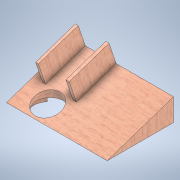
# Autodesk Inventor part: CAP PROCESS SKETCH
Saved by Autodesk Inventor 2021 (Build 250183000, 183)
## iProperties
Created: 2021-07-15
Part Number: CAP PROCESS SKETCH
Material: Generic
Document SubType Name: Modeling
Designer: HP
Density: 1 g/cm^3
Appearance: Plywood - Weathered
Author: HP
Autodesk Inventor part; units mm, degrees
ref_plane "YZ Plane" through (0, 0, 0) normal (1, 0, 0) x (0, 1, 0)
ref_plane "XZ Plane" through (0, 0, 0) normal (0, 1, 0) x (-1, 0, 0)
ref_plane "XY Plane" through (0, 0, 0) normal (0, 0, 1) x (1, 0, 0)
sketch "Sketch1" plane through (0, 0, 0) normal (1, 0, 0) x (0, 1, 0)
  line L0 (0, 0) -> (25.4, 0)
  line L1 (0, 0) -> (0, 75.184)
  line L2 (0, 75.184) -> (25.4, 0)
  dimension "d0" = 25.4
  dimension "d1" = 75.184
  constraints: 6 end point, 1 horizontal, 1 vertical
  measures "d0" distance of L0.start L0.end
  measures "d1" distance of L0.start L1.end
extrude "Extrusion1" add sketch "Sketch1" along normal blind 114.3
sketch "Sketch2" plane through (0, 0, 75.184) normal (0, 0.9473953, 0.320066) x (1, 0, 0)
  circle A0 centre (30.1625, 17.4625) radius 13.4874
  point P0 (0, 71.229)
  dimension "d4" = 26.9748
  constraints: 1 centre point
  measures "d4" diameter of A0
extrude "Extrusion2" add sketch "Sketch2" along normal blind 25.4
sketch "Sketch3" plane through (30.1625, 29.653, 66.7698) normal (0, 0.9473953, 0.320066) x (1, 0, 0)
  circle A0 centre (0, 0) radius 14.9075
  point P0 (-30.1625, 53.7665)
  constraints: 1 centre point
extrude "Extrusion3" cut sketch "Sketch3" against normal blind 76.2
sketch "Sketch4" plane through (0, 0, 0) normal (0, -1, 0) x (1, 0, 0)
  point P0 (0, 0)
sketch "Sketch5" plane through (0, 0, 0) normal (0, -1, 0) x (1, 0, 0)
  arc A0 (42.3045, 45.008) -> (44.45, 66.675) centre (30.1625, 57.15) ccw
  arc A1 (44.3808, 43.1924) -> (47.2504, 67.396) centre (30.1625, 57.15) ccw
  arc A2 (15.875, 66.675) -> (17.0779, 46.0302) centre (30.1625, 57.15) ccw
  arc A3 (13.625, 68.2625) -> (14.8563, 44.3948) centre (30.1625, 57.15) ccw
  line L0 (13.625, 68.2625) -> (15.875, 66.675)
  line L1 (14.8563, 44.3948) -> (17.0779, 46.0302)
  line L2 (44.45, 66.675) -> (47.2504, 67.396)
  line L3 (42.3045, 45.008) -> (44.3808, 43.1924)
  point P0 (0, 0)
  constraints: 8 end point, 8 point on circle, 4 centre point, 3 coincident
extrude "Extrusion4" add sketch "Sketch5" along normal blind 5.08
sketch "Sketch6" plane through (0, 0, 75.184) normal (0, 0.9473953, 0.320066) x (1, 0, 0)
  line L0 (0, 79.3586) -> (114.3, 79.3586) projected
  line L1 (14.2875, 31.75) -> (11.1125, 31.75)
  line L2 (11.1125, 31.75) -> (11.1125, 79.3586)
  line L3 (11.1125, 79.3586) -> (14.2875, 79.3586)
  line L4 (14.2875, 79.3586) -> (14.2875, 31.75)
  line L5 (49.2743, 31.75) -> (45.5103, 31.75)
  line L6 (45.5103, 31.75) -> (45.5103, 79.375)
  line L7 (45.5103, 79.375) -> (49.2743, 79.375)
  line L8 (49.2743, 79.375) -> (49.2743, 31.75)
  point P0 (0, 71.229)
  constraints: 16 end point, 4 parallel, 2 horizontal, 2 perpendicular, 2 point on line
extrude "Extrusion5" add sketch "Sketch6" along normal blind 25.4
body "Solid1"
